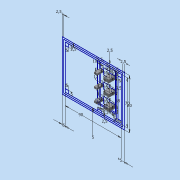
# Autodesk Inventor part: Top
Saved by Autodesk Inventor 2015 (Build 190159000, 159)
## iProperties
Created: 2014-12-25
Part Number: Top
Material: Generic
Document SubType Name: Modeling
Designer: Openlab
Density: 1 g/cm^3
Appearance: Default
Author: Openlab
Autodesk Inventor part; units mm, degrees
ref_plane "YZ Plane" through (0, 0, 0) normal (1, 0, 0) x (0, 1, 0)
ref_plane "XZ Plane" through (0, 0, 0) normal (0, 1, 0) x (-1, 0, 0)
ref_plane "XY Plane" through (0, 0, 0) normal (0, 0, 1) x (1, 0, 0)
sketch "Sketch1" plane through (0, 0, 0) normal (0, 1, 0) x (-1, 0, 0)
  line L0 (100, 0) -> (0, 0)
  line L1 (0, 0) -> (0, -80)
  line L2 (0, -80) -> (100, -80)
  line L3 (100, -80) -> (100, 0)
  line L4 (95, -5) -> (68, -5)
  line L5 (5, -5) -> (5, -75)
  line L6 (5, -75) -> (95, -75)
  line L7 (95, -75) -> (95, -5)
  line L8 (33.5, -10) -> (23.5, -10)
  line L9 (23.5, -10) -> (23.5, -20)
  line L10 (23.5, -20) -> (33.5, -20)
  line L11 (95, -65) -> (95, -5)
  line L12 (23.5, -50) -> (23.5, -60)
  line L13 (23.5, -60) -> (33.5, -60)
  line L14 (33.5, -50) -> (23.5, -50)
  line L15 (95, -5) -> (90, -5)
  line L16 (90, -5) -> (90, -10)
  line L17 (90, -10) -> (95, -10)
  line L18 (95, -10) -> (95, -5)
  line L19 (95, -75) -> (90, -75)
  line L20 (90, -75) -> (90, -70)
  line L21 (90, -70) -> (95, -70)
  line L22 (95, -70) -> (95, -75)
  line L23 (5, -5) -> (10, -5)
  line L24 (10, -5) -> (10, -10)
  line L25 (10, -10) -> (5, -10)
  line L26 (5, -10) -> (5, -5)
  line L27 (5, -75) -> (10, -75)
  line L28 (10, -75) -> (10, -70)
  line L29 (10, -70) -> (5, -70)
  line L30 (5, -70) -> (5, -75)
  line L31 (95, -5) -> (68, -5)
  line L32 (14.5, -63) -> (14.5, -5)
  line L33 (38.5, -63) -> (14.5, -63)
  line L34 (14.5, -5) -> (5, -5)
  line L35 (23.5, -40) -> (33.5, -40)
  line L36 (23.5, -30) -> (23.5, -40)
  line L37 (33.5, -30) -> (23.5, -30)
  line L38 (33.5, -60) -> (33.5, -56.5)
  line L39 (33.5, -53.5) -> (33.5, -50)
  line L40 (38.5, -56.5) -> (38.5, -63)
  line L41 (33.5, -56.5) -> (38.5, -56.5)
  line L42 (38.5, -53.5) -> (33.5, -53.5)
  line L43 (33.5, -40) -> (33.5, -36.5)
  line L44 (33.5, -33.5) -> (33.5, -30)
  line L45 (38.5, -36.5) -> (38.5, -53.5)
  line L46 (33.5, -20) -> (33.5, -16.5)
  line L47 (33.5, -13.5) -> (33.5, -10)
  line L48 (38.5, -5) -> (38.5, -13.5)
  line L49 (38.5, -16.5) -> (38.5, -33.5)
  line L50 (38.5, -36.5) -> (33.5, -36.5)
  line L51 (38.5, -33.5) -> (33.5, -33.5)
  line L52 (33.5, -16.5) -> (38.5, -16.5)
  line L53 (33.5, -13.5) -> (38.5, -13.5)
  line L54 (33.5, -56.5) -> (33.5, -53.5)
  line L55 (38.5, -56.5) -> (38.5, -53.5)
  line L56 (38.5, -36.5) -> (38.5, -33.5)
  line L57 (33.5, -36.5) -> (33.5, -33.5)
  line L58 (33.5, -16.5) -> (33.5, -13.5)
  line L59 (38.5, -16.5) -> (38.5, -13.5)
  line L60 (14.5, -57.5) -> (23.5, -57.5)
  line L61 (14.5, -52.5) -> (23.5, -52.5)
  line L62 (14.5, -37.5) -> (23.5, -37.5)
  line L63 (14.5, -32.5) -> (23.5, -32.5)
  line L64 (14.5, -17.5) -> (23.5, -17.5)
  line L65 (14.5, -12.5) -> (23.5, -12.5)
  line L66 (40, -5) -> (40, -63)
  line L67 (68, -5) -> (43, -5)
  line L68 (40, -5) -> (38.5, -5)
  line L69 (37, -75) -> (37, -72)
  line L70 (40, -5) -> (43, -5)
  line L71 (13, -5) -> (13, -72)
  line L72 (13, -72) -> (14.5, -72)
  line L73 (14.5, -72) -> (14.5, -75)
  line L74 (2.5002, -77.5) -> (2.5002, -2.5)
  line L75 (2.5002, -2.5) -> (97.5, -2.5)
  line L76 (97.5, -2.5) -> (97.5, -77.5)
  line L77 (97.5, -77.5) -> (2.5002, -77.5)
  line L78 (40, -63) -> (43, -63)
  line L79 (43, -75) -> (43, -72)
  line L80 (43, -63) -> (43, -5)
  line L81 (43, -72) -> (37, -72)
  line L82 (13.5, -5) -> (13.5, -65)
  line L83 (13.5, -65) -> (43.5, -65)
  line L84 (43.5, -65) -> (43.5, -5)
  line L85 (14.5, -5) -> (38.5, -5)
  line L86 (10, -75) -> (10, -5)
  dimension "d0" = 5
  dimension "d1" = 5
  dimension "d2" = 5
  dimension "d4" = 10
  dimension "d5" = 10
  dimension "d6" = 10
  dimension "d7" = 10
  dimension "d8" = 70
  dimension "d9" = 5
  dimension "d10" = 5
  dimension "d11" = 5
  dimension "d12" = 5
  dimension "d13" = 5
  dimension "d14" = 5
  dimension "d15" = 5
  dimension "d16" = 5
  dimension "d19" = 90
  dimension "d20" = 9.5
  dimension "d21" = 3
  dimension "d22" = 10
  dimension "d23" = 80
  dimension "d24" = 10
  dimension "d25" = 10
  dimension "d26" = 10
  dimension "d27" = 10
  dimension "d30" = 6.5
  dimension "d47" = 17
  dimension "d54" = 5
  dimension "d55" = 2.5
  dimension "d56" = 5
  dimension "d57" = 2.5
  dimension "d58" = 5
  dimension "d59" = 2.5
  dimension "d60" = 1.5
  dimension "d61" = 9
  dimension "d62" = 58
  dimension "d63" = 1.5
  dimension "d65" = 3
  dimension "d67" = 2.5002
  dimension "d68" = 2.5
  dimension "d69" = 2.5
  dimension "d70" = 2.5
  dimension "d71" = 3
  dimension "d72" = 6
  dimension "d73" = 3
  dimension "d74" = 2.5
  dimension "d75" = 24
  dimension "d76" = 3
  dimension "d77" = 3
  dimension "d78" = 3
  dimension "d79" = 17
  dimension "d88" = 10
  dimension "d90" = 10
  dimension "d91" = 5
  constraints: 174 end point, 35 parallel, 35 perpendicular, 17 horizontal, 17 point on line, 11 collinear, 6 vertical, 2 coincident
  measures "d0" distance between parallel lines of L2 L6
  measures "d1" distance between parallel lines of L7 L3
  measures "d2" distance between parallel lines of L1 L5
  measures "d4" distance of L10.end L8.start
  measures "d5" distance of L9.end L10.end
  measures "d6" distance of L13.end L14.start
  measures "d7" distance of L12.end L13.end
  measures "d8" distance of L5.start L5.end
  measures "d9" distance of L17.end L16.end
  measures "d10" distance of L16.end L15.end
  measures "d11" distance of L20.end L21.end
  measures "d12" distance of L19.end L20.end
  measures "d13" distance of L24.end L25.end
  measures "d14" distance of L23.end L24.end
  measures "d15" distance of L29.end L28.end
  measures "d16" distance of L28.end L27.end
  measures "d19" distance of L5.end L6.end
  measures "d20" distance between parallel lines of L5 L32
  measures "d21" distance between parallel lines of L33 L13
  measures "d22" distance between parallel lines of L0 L8
  measures "d23" distance between parallel lines of L0 L2
  measures "d24" distance of L35.end L37.start
  measures "d25" distance of L35.start L35.end
  measures "d26" distance between parallel lines of L37 L10
  measures "d27" distance between parallel lines of L14 L35
  measures "d30" distance of L40.start L33.start
  measures "d47" distance of L42.start L45.start
  measures "d54" distance between parallel lines of L65 L64
  measures "d55" distance between parallel lines of L8 L65
  measures "d56" distance between parallel lines of L63 L62
  measures "d57" distance between parallel lines of L37 L63
  measures "d58" distance between parallel lines of L60 L61
  measures "d59" distance between parallel lines of L14 L61
  measures "d60" distance between parallel lines of L66 L48
  measures "d61" distance between parallel lines of L12 L32
  measures "d62" distance of L32.start L32.end
  measures "d63" distance between parallel lines of L32 L71
  measures "d65" distance of L69.start L69.end
  measures "d67" distance between parallel lines of L1 L74
  measures "d68" distance between parallel lines of L0 L75
  measures "d69" distance between parallel lines of L2 L77
  measures "d70" distance between parallel lines of L3 L76
  measures "d71" distance of L66.end L78.end
  measures "d72" distance of L79.end L69.end
  measures "d73" distance of L72.end L73.end
  measures "d74" distance between parallel lines of L75 L4
  measures "d75" distance of L33.start L32.start
  measures "d76" distance of L40.start L42.start
  measures "d77" distance of L45.start L49.end
  measures "d78" distance of L49.start L48.end
  measures "d79" distance between parallel lines of L51 L52
  measures "d88" distance between parallel lines of L84 L47
  measures "d90" distance between parallel lines of L82 L9
  measures "d91" distance between parallel lines of L83 L13
extrude "Extrusion5" [suppressed]
extrude "Extrusion6" [suppressed]
extrude "Extrusion7" add sketch "Sketch1" against normal blind 10 contours L59 L52 L58 L53 | L65 L9 L64 L32 | L56 L50 L57 L51 | L63 L36 L62 L32 | L55 L41 L54 L42 | L61 L12 L60 L32
body "Solid2"
